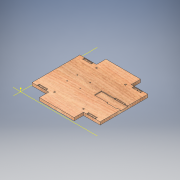
# Autodesk Inventor part: BottomPlate
Saved by Autodesk Inventor 2017 (Build 210142000, 142)
## iProperties
Created: 2017-01-25
Part Number: BottomPlate
Material: Wood (Oak)
Document SubType Name: Modeling
Designer: Naga
Density: 0.76 g/cm^3
Appearance: Birch - Natural Polished
Author: Naga
Autodesk Inventor part; units mm, degrees
ref_plane "YZ Plane" through (0, 0, 0) normal (1, 0, 0) x (0, 1, 0)
ref_plane "XY Plane" through (0, 0, 0) normal (0, 0, 1) x (1, 0, 0)
sketch "Sketch2" plane through (0, 0, 0) normal (0, 1, 0) x (-1, 0, 0)
  line L0 (0, 0) -> (-304.8, 0) construction
  line L1 (-304.8, 0) -> (-304.8, -304.8) construction
  line L2 (-304.8, -304.8) -> (0, -304.8) construction
  line L3 (0, -304.8) -> (0, 0) construction
  line L4 (-193.35, -166.5986) -> (-296.45, -166.5986)
  line L5 (-298.45, -140.1986) -> (-298.45, -164.5986)
  line L6 (-296.45, -138.1986) -> (-193.35, -138.1986)
  arc A0 (-193.35, -166.3986) -> (-193.35, -138.3986) centre (-201.35, -152.3986) ccw
  line L7 (-279.4, -254.74) -> (-279.4, -248.24) construction
  line L8 (-242.6, -254.74) -> (-242.6, -248.24) construction
  circle A1 centre (-246.2, -251.49) radius 1.25
  circle A2 centre (-275.8, -251.49) radius 1.25
  line L9 (-279.4, -254.74) -> (-242.6, -254.74) construction
  line L10 (-62.2, -254.74) -> (-25.4, -254.74) construction
  line L11 (-25.4, -254.74) -> (-25.4, -248.24) construction
  circle A3 centre (-29, -251.49) radius 1.25
  circle A4 centre (-58.6, -251.49) radius 1.25
  line L12 (-62.2, -254.74) -> (-62.2, -248.24) construction
  circle A5 centre (-29, -53.4043) radius 1.25
  circle A6 centre (-58.6, -53.4043) radius 1.25
  line L13 (-242.6, -50.1543) -> (-242.6, -56.6543) construction
  line L14 (-279.4, -50.1543) -> (-279.4, -56.6543) construction
  circle A7 centre (-275.8, -53.4043) radius 1.25
  circle A8 centre (-246.2, -53.4043) radius 1.25
  line L15 (-242.6, -56.6543) -> (-279.4, -56.6543) construction
  line L16 (-62.2, -248.24) -> (-25.4, -248.24) construction
  line L17 (-279.4, -248.24) -> (-242.6, -248.24) construction
  circle A9 centre (-130.78, -175.0162) radius 1.778
  circle A10 centre (-73.63, -175.0162) radius 1.778
  circle A11 centre (-73.63, -130.8202) radius 1.778
  circle A12 centre (-130.78, -130.8202) radius 1.778
  circle A13 centre (-43.8, -251.49) radius 1.25
  circle A14 centre (-43.8, -53.4043) radius 1.25
  circle A15 centre (-261, -53.4043) radius 1.25
  circle A16 centre (-261, -251.49) radius 1.25
  line L18 (-76.2, -6.35) -> (-228.6, -6.35)
  line L19 (-228.6, -298.45) -> (-76.2, -298.45)
  line L20 (-76.2, -6.35) -> (-228.6, -298.45) construction
  line L21 (-228.6, -6.35) -> (-76.2, -298.45) construction
  line L22 (-301.625, -47.625) -> (-301.625, -257.175)
  line L23 (-3.175, -257.175) -> (-3.175, -47.625)
  line L24 (-3.175, -47.625) -> (-301.625, -257.175) construction
  line L25 (-301.625, -47.625) -> (-3.175, -257.175) construction
  line L26 (-88.9, -257.175) -> (-88.9, -244.475)
  line L27 (-88.9, -244.475) -> (-85.725, -244.475)
  circle A17 centre (-88.9, -244.475) radius 3.175
  line L28 (-88.9, -244.475) -> (-215.9, -244.475)
  line L29 (-215.9, -244.475) -> (-215.9, -60.325) construction
  line L30 (-215.9, -60.325) -> (-88.9, -244.475) construction
  line L31 (-88.9, -60.325) -> (-215.9, -244.475) construction
  circle A18 centre (-215.9, -244.475) radius 3.175
  circle A19 centre (-88.9, -60.325) radius 3.175
  circle A20 centre (-215.9, -60.325) radius 3.175
  line L32 (-76.2, -298.45) -> (-76.2, -257.175)
  line L33 (-76.2, -47.625) -> (-76.2, -6.35)
  line L34 (-3.175, -47.625) -> (-76.2, -47.625)
  line L35 (-228.6, -47.625) -> (-301.625, -47.625)
  line L36 (-88.9, -60.325) -> (-88.9, -63.5)
  line L37 (-88.9, -241.3) -> (-88.9, -244.475)
  line L38 (-215.9, -60.325) -> (-200.4391, -60.325)
  line L39 (-104.3609, -60.325) -> (-88.9, -60.325)
  line L40 (-228.6, -6.35) -> (-228.6, -47.625)
  line L41 (-228.6, -138.1986) -> (-228.6, -166.5986)
  line L42 (-228.6, -257.175) -> (-228.6, -298.45)
  line L43 (-301.625, -257.175) -> (-228.6, -257.175)
  line L44 (-97.7348, -257.175) -> (-88.9, -257.175)
  line L45 (-76.2, -257.175) -> (-3.175, -257.175)
  line L46 (-76.2, -244.475) -> (-76.2, -248.24)
  point P0 (-152.4, -152.4)
  dimension "d8" = 304.8
  dimension "d9" = 304.8
  dimension "d10" = 152.4
  dimension "d11" = 292.1
  dimension "d12" = 298.45
  dimension "d13" = 209.55
  dimension "d14" = 12.7
  dimension "d15" = 12.7
  dimension "d16" = 6.35
  dimension "d17" = 127
  dimension "d18" = 184.15
  constraints: 94 end point, 21 parallel, 20 centre point, 10 perpendicular, 7 horizontal, 6 midpoint, 6 point on line, 4 point on circle, 1 coincident, 1 vertical, 1 vertical alignment, 8 other
  measures "d8" distance of L2.end L1.end
  measures "d9" distance of L1.end L0.end
  measures "d10" distance of L19.end L19.start
  measures "d11" distance of L19.start L18.end
  measures "d12" distance of L23.start L22.end
  measures "d13" distance of L22.end L22.start
  measures "d14" distance of L46.start L26.end
  measures "d15" distance of L26.start L26.end
  measures "d16" diameter of A17
  measures "d17" distance of L28.start A18.centre
  measures "d18" distance of L28.start point (-88.9, -60.325)
extrude "Extrusion1" add sketch "Sketch2" along normal blind 12.7
ref_plane "Work Plane1" through (0, 12.7, 0) normal (0, 1, 0) x (-1, 0, 0)
sketch "Sketch6" plane through (0, 12.7, 0) normal (0, 1, 0) x (-1, 0, 0)
  line L0 (0, 0) -> (-304.8, 0)
  line L1 (-304.8, 0) -> (-304.8, -304.8)
  line L2 (-304.8, -304.8) -> (0, -304.8)
  line L3 (0, -304.8) -> (0, 0)
  line L4 (-76.2, -6.35) -> (-228.6, -6.35)
  line L5 (-228.6, -6.35) -> (-228.6, -298.45)
  line L6 (-228.6, -298.45) -> (-76.2, -298.45)
  line L7 (-76.2, -298.45) -> (-76.2, -6.35)
  line L8 (-76.2, -6.35) -> (-228.6, -298.45) construction
  line L9 (-228.6, -6.35) -> (-76.2, -298.45) construction
  line L10 (-3.175, -47.625) -> (-301.625, -47.625)
  line L11 (-301.625, -47.625) -> (-301.625, -257.175)
  line L12 (-301.625, -257.175) -> (-3.175, -257.175)
  line L13 (-3.175, -257.175) -> (-3.175, -47.625)
  line L14 (-3.175, -47.625) -> (-301.625, -257.175) construction
  line L15 (-301.625, -47.625) -> (-3.175, -257.175) construction
  line L16 (-76.2, -257.175) -> (-88.9, -257.175)
  line L17 (-88.9, -257.175) -> (-88.9, -244.475)
  line L18 (-88.9, -244.475) -> (-76.2, -244.475)
  line L19 (-76.2, -244.475) -> (-76.2, -257.175)
  circle A0 centre (-88.9, -244.475) radius 3.175
  line L20 (-215.9, -60.325) -> (-88.9, -60.325)
  line L21 (-88.9, -60.325) -> (-88.9, -244.475)
  line L22 (-88.9, -244.475) -> (-215.9, -244.475)
  line L23 (-215.9, -244.475) -> (-215.9, -60.325)
  line L24 (-215.9, -60.325) -> (-88.9, -244.475) construction
  line L25 (-88.9, -60.325) -> (-215.9, -244.475) construction
  circle A1 centre (-215.9, -244.475) radius 3.175
  circle A2 centre (-88.9, -60.325) radius 3.175
  circle A3 centre (-215.9, -60.325) radius 3.175
  circle A4 centre (-261, -53.4043) radius 1.25 projected
  line L26 (-241.95, -57.5318) -> (-280.05, -57.5318)
  line L27 (-280.05, -57.5318) -> (-280.05, -49.2768)
  line L28 (-280.05, -49.2768) -> (-241.95, -49.2768)
  line L29 (-241.95, -49.2768) -> (-241.95, -57.5318)
  line L30 (-241.95, -57.5318) -> (-280.05, -49.2768) construction
  line L31 (-280.05, -57.5318) -> (-241.95, -49.2768) construction
  circle A5 centre (-261, -251.49) radius 1.25 projected
  circle A6 centre (-43.8, -251.49) radius 1.25 projected
  circle A7 centre (-43.8, -53.4043) radius 1.25 projected
  line L32 (-152.4, -152.4) -> (-301.625, -152.4)
  line L33 (-301.625, -152.4) -> (-187.325, -152.4)
  line L34 (-301.625, -152.4) -> (-301.625, -136.525)
  line L35 (-301.625, -47.625) -> (-301.625, -257.175) projected
  line L36 (-301.625, -136.525) -> (-187.325, -136.525)
  line L37 (-187.325, -136.525) -> (-187.325, -168.275)
  line L38 (-187.325, -168.275) -> (-301.625, -168.275)
  line L39 (-301.625, -168.275) -> (-301.625, -136.525)
  line L40 (-241.95, -255.6175) -> (-280.05, -255.6175)
  line L41 (-280.05, -255.6175) -> (-280.05, -247.3625)
  line L42 (-280.05, -247.3625) -> (-241.95, -247.3625)
  line L43 (-241.95, -247.3625) -> (-241.95, -255.6175)
  circle A8 centre (-261, -251.49) radius 1.25 projected
  line L44 (-241.95, -255.6175) -> (-280.05, -247.3625) construction
  line L45 (-280.05, -255.6175) -> (-241.95, -247.3625) construction
  line L46 (-24.75, -255.6175) -> (-62.85, -255.6175)
  line L47 (-62.85, -255.6175) -> (-62.85, -247.3625)
  line L48 (-62.85, -247.3625) -> (-24.75, -247.3625)
  line L49 (-24.75, -247.3625) -> (-24.75, -255.6175)
  line L50 (-24.75, -255.6175) -> (-62.85, -247.3625) construction
  line L51 (-62.85, -255.6175) -> (-24.75, -247.3625) construction
  line L52 (-24.75, -49.2768) -> (-62.85, -49.2768)
  line L53 (-62.85, -49.2768) -> (-62.85, -57.5318)
  line L54 (-62.85, -57.5318) -> (-24.75, -57.5318)
  line L55 (-24.75, -57.5318) -> (-24.75, -49.2768)
  circle A9 centre (-43.8, -53.4043) radius 1.25 projected
  line L56 (-24.75, -49.2768) -> (-62.85, -57.5318) construction
  line L57 (-62.85, -49.2768) -> (-24.75, -57.5318) construction
  dimension "d49" = 304.8
  dimension "d50" = 304.8
  dimension "d51" = 152.4
  dimension "d52" = 292.1
  dimension "d53" = 298.45
  dimension "d54" = 209.55
  dimension "d55" = 12.7
  dimension "d56" = 12.7
  dimension "d57" = 6.35
  dimension "d58" = 127
  dimension "d59" = 184.15
  dimension "d62" = 38.1
  dimension "d63" = 8.255
  dimension "d64" = 114.3
  dimension "d65" = 15.875
  dimension "d66" = 31.75
  dimension "d67" = 8.255
  dimension "d68" = 38.1
  constraints: 114 end point, 20 parallel, 15 midpoint, 11 horizontal, 10 perpendicular, 6 point on line, 4 centre point, 1 coincident, 1 vertical, 6 other
  measures "d49" distance of L2.end L1.end
  measures "d50" distance of L1.end L0.end
  measures "d51" distance of L6.end L5.end
  measures "d52" distance of L5.end L4.end
  measures "d53" distance of L12.end L11.end
  measures "d54" distance of L11.end L10.end
  measures "d55" distance of L17.end L18.end
  measures "d56" distance of L16.end L17.end
  measures "d57" diameter of A0
  measures "d58" distance of L21.end A1.centre
  measures "d59" distance of L21.end A2.centre
  measures "d62" distance of L27.end L28.end
  measures "d63" distance of L26.end L27.end
  measures "d64" distance of L32.end L33.end
  measures "d65" distance of L32.end L34.end
  measures "d66" distance of L36.end L37.end
  measures "d67" distance of L40.end L41.end
  measures "d68" distance of L47.end L48.end
extrude "Extrusion2" cut sketch "Sketch6" against normal blind 3.175 contours L26 L27 L28 L29 | L40 L41 L42 L43 | L46 L47 L48 L49 | L55 L54 L53 L52
sketch "Sketch7" plane through (0, 12.7, 0) normal (0, 1, 0) x (1, 0, 0)
  line L0 (24.75, 247.3625) -> (24.75, 255.6175) projected
  line L1 (24.75, 255.6175) -> (62.85, 255.6175) projected
  line L2 (62.85, 255.6175) -> (62.85, 247.3625) projected
  line L3 (62.85, 247.3625) -> (24.75, 247.3625) projected
  line L4 (241.95, 49.2768) -> (241.95, 57.5318) projected
  line L5 (241.95, 57.5318) -> (280.05, 57.5318) projected
  line L6 (280.05, 57.5318) -> (280.05, 49.2768) projected
  line L7 (280.05, 49.2768) -> (241.95, 49.2768) projected
  line L8 (241.95, 247.3625) -> (241.95, 255.6175) projected
  line L9 (241.95, 255.6175) -> (280.05, 255.6175) projected
  line L10 (280.05, 255.6175) -> (280.05, 247.3625) projected
  line L11 (280.05, 247.3625) -> (241.95, 247.3625) projected
  line L12 (62.85, 57.5318) -> (62.85, 49.2768) projected
  line L13 (62.85, 49.2768) -> (24.75, 49.2768) projected
  line L14 (24.75, 49.2768) -> (24.75, 57.5318) projected
  line L15 (24.75, 57.5318) -> (62.85, 57.5318) projected
  circle A0 centre (88.9, 244.475) radius 3.175 projected
  circle A1 centre (215.9, 60.325) radius 3.175 projected
  circle A2 centre (88.9, 60.325) radius 3.175 projected
  circle A3 centre (215.9, 244.475) radius 3.175 projected
  circle A4 centre (130.78, 130.8202) radius 1.778 projected
  circle A5 centre (73.63, 130.8202) radius 1.778 projected
  circle A6 centre (73.63, 175.0162) radius 1.778 projected
  circle A7 centre (130.78, 175.0162) radius 1.778 projected
  line L16 (76.2, 6.35) -> (228.6, 6.35) projected
  line L17 (228.6, 6.35) -> (228.6, 47.625) projected
  line L18 (228.6, 47.625) -> (301.625, 47.625) projected
  line L19 (301.625, 47.625) -> (301.625, 257.175) projected
  line L20 (301.625, 257.175) -> (228.6, 257.175) projected
  line L21 (228.6, 257.175) -> (228.6, 298.45) projected
  line L22 (228.6, 298.45) -> (76.2, 298.45) projected
  line L23 (76.2, 298.45) -> (76.2, 257.175) projected
  line L24 (76.2, 257.175) -> (3.175, 257.175) projected
  line L25 (3.175, 257.175) -> (3.175, 47.625) projected
  line L26 (3.175, 47.625) -> (76.2, 47.625) projected
  line L27 (76.2, 47.625) -> (76.2, 6.35) projected
  line L28 (301.625, 47.625) -> (301.625, 257.175) projected
  line L29 (301.625, 152.4) -> (187.325, 152.4)
  line L30 (244.475, 152.4) -> (244.475, 168.275)
  line L31 (187.325, 136.525) -> (301.625, 136.525)
  line L32 (301.625, 136.525) -> (301.625, 168.275)
  line L33 (301.625, 168.275) -> (187.325, 168.275)
  line L34 (187.325, 168.275) -> (187.325, 136.525)
  line L35 (187.325, 136.525) -> (301.625, 168.275) construction
  line L36 (301.625, 136.525) -> (187.325, 168.275) construction
  line L37 (244.475, 168.275) -> (252.73, 168.275)
  line L38 (252.73, 168.275) -> (252.73, 171.45)
  line L39 (252.73, 171.45) -> (244.475, 171.45)
  line L40 (244.475, 171.45) -> (244.475, 168.275)
  line L41 (244.475, 169.8625) -> (252.73, 169.8625) construction
  line L42 (246.0625, 168.275) -> (251.1425, 168.275)
  line L43 (251.1425, 171.45) -> (246.0625, 171.45)
  arc A8 (246.0625, 171.45) -> (246.0625, 168.275) centre (246.0625, 169.8625) ccw
  arc A9 (251.1425, 168.275) -> (251.1425, 171.45) centre (251.1425, 169.8625) ccw
  arc A10 (270.1925, 168.275) -> (270.1925, 171.45) centre (270.1925, 169.8625) ccw
  line L44 (265.1125, 168.275) -> (270.1925, 168.275)
  line L45 (270.1925, 171.45) -> (265.1125, 171.45)
  arc A11 (265.1125, 171.45) -> (265.1125, 168.275) centre (265.1125, 169.8625) ccw
  arc A12 (289.2425, 168.275) -> (289.2425, 171.45) centre (289.2425, 169.8625) ccw
  line L46 (284.1625, 168.275) -> (289.2425, 168.275)
  line L47 (289.2425, 171.45) -> (284.1625, 171.45)
  arc A13 (284.1625, 171.45) -> (284.1625, 168.275) centre (284.1625, 169.8625) ccw
  arc A14 (251.1425, 133.35) -> (251.1425, 136.525) centre (251.1425, 134.9375) ccw
  line L48 (246.0625, 133.35) -> (251.1425, 133.35)
  line L49 (251.1425, 136.525) -> (246.0625, 136.525)
  arc A15 (246.0625, 136.525) -> (246.0625, 133.35) centre (246.0625, 134.9375) ccw
  arc A16 (270.1925, 133.35) -> (270.1925, 136.525) centre (270.1925, 134.9375) ccw
  line L50 (265.1125, 133.35) -> (270.1925, 133.35)
  line L51 (270.1925, 136.525) -> (265.1125, 136.525)
  arc A17 (265.1125, 136.525) -> (265.1125, 133.35) centre (265.1125, 134.9375) ccw
  arc A18 (289.2425, 133.35) -> (289.2425, 136.525) centre (289.2425, 134.9375) ccw
  line L52 (284.1625, 133.35) -> (289.2425, 133.35)
  line L53 (289.2425, 136.525) -> (284.1625, 136.525)
  arc A19 (284.1625, 136.525) -> (284.1625, 133.35) centre (284.1625, 134.9375) ccw
  point P0 (0, 0)
  point P1 (248.6025, 169.8625)
  dimension "d71" = 114.3
  dimension "d72" = 15.875
  dimension "d73" = 8.255
  dimension "d74" = 3.175
  dimension "d77" = 19.05
  dimension "d80" = 34.925
  constraints: 52 end point, 26 point on circle, 12 centre point, 7 midpoint, 5 parallel, 4 horizontal, 4 tangent, 3 point on line, 2 perpendicular, 2 vertical, 50 other
  measures "d71" distance of L29.start L29.end
  measures "d72" distance of L30.start L30.end
  measures "d73" distance of L39.end L38.end
  measures "d74" distance of L38.end L37.end
  measures "d77" distance of A9.centre A10.centre
  measures "d80" distance of A9.centre A14.centre
extrude "Extrusion3" cut sketch "Sketch7" against normal up to surface (12.7 mm away) contours A18 L52 A19 L31 | L33 A13 L47 A12 | A16 L50 A17 L31 | A8 L39 A9 L33 | L33 A11 L45 A10 | L31 A14 L48 A15
sketch "Sketch8" plane through (0, 12.7, 0) normal (0, 1, 0) x (1, 0, 0)
  line L0 (301.625, 47.625) -> (301.625, 257.175) projected
  line L1 (301.625, 152.4) -> (187.325, 152.4)
  line L2 (301.625, 152.4) -> (415.925, 152.4) construction
  line L3 (244.475, 152.4) -> (244.475, 168.275)
  line L4 (187.325, 136.525) -> (301.625, 136.525)
  line L5 (301.625, 136.525) -> (301.625, 168.275)
  line L6 (301.625, 168.275) -> (187.325, 168.275)
  line L7 (187.325, 168.275) -> (187.325, 136.525)
  line L8 (187.325, 136.525) -> (301.625, 168.275) construction
  line L9 (301.625, 136.525) -> (187.325, 168.275) construction
  point P0 (0, 0)
  dimension "d85" = 114.3
  dimension "d86" = 180
  constraints: 18 end point, 4 midpoint, 3 horizontal, 2 parallel, 1 collinear, 1 perpendicular, 1 point on line, 1 vertical
  measures "d85" distance of L1.start L1.end
  measures "d86" angle of L1 L2
extrude "Extrusion4" cut sketch "Sketch8" against normal blind 3.175
sketch "Sketch9" plane through (0, 12.7, 0) normal (0, 1, 0) x (1, 0, 0)
  point P0 (0, 0)
sketch "Sketch10" plane through (0, 12.7, 0) normal (0, 1, 0) x (1, 0, 0)
  arc A0 (251.1425, 133.35) -> (251.1425, 136.525) centre (251.1425, 134.9375) ccw projected
  line L0 (251.1425, 136.525) -> (284.1625, 136.525)
  line L1 (284.1625, 136.525) -> (284.1625, 133.35)
  line L2 (284.1625, 133.35) -> (251.1425, 133.35)
  arc A1 (284.1625, 136.525) -> (284.1625, 133.35) centre (284.1625, 134.9375) ccw projected
  line L3 (251.1425, 133.35) -> (251.1425, 136.525)
  line L4 (301.625, 47.625) -> (301.625, 257.175) projected
  line L5 (301.625, 152.4) -> (290.5314, 152.4)
  line L6 (251.1425, 168.275) -> (284.1625, 168.275)
  line L7 (284.1625, 168.275) -> (284.1625, 171.45)
  line L8 (284.1625, 171.45) -> (251.1425, 171.45)
  line L9 (251.1425, 171.45) -> (251.1425, 168.275)
  point P0 (0, 0)
  point P1 (251.1425, 169.8625)
  dimension "d10" = 152.4
  dimension "d11" = 292.1
  dimension "d12" = 298.45
  dimension "d13" = 209.55
  dimension "d14" = 12.7
  dimension "d15" = 12.7
  dimension "d16" = 6.35
  dimension "d17" = 127
  dimension "d18" = 184.15
  constraints: 18 end point, 6 symmetric about line, 2 horizontal, 2 perpendicular, 2 tangent, 1 midpoint
extrude "Extrusion5" cut sketch "Sketch10" against normal up to surface (12.7 mm away)
body "Solid1"
